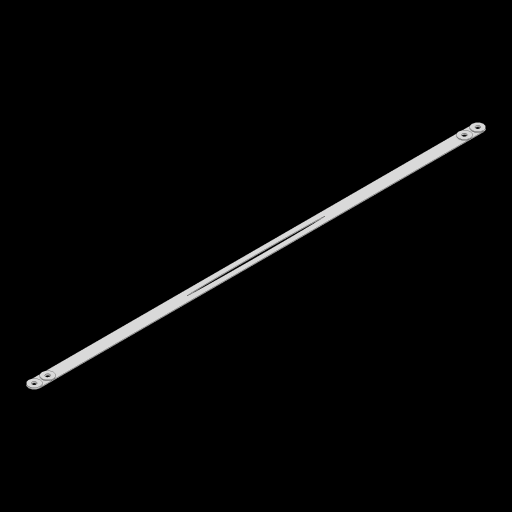
# Autodesk Inventor part: szalag4
Saved by Autodesk Inventor 2023 (Build 270158000, 158)
## iProperties
Created: 2022-11-17
Part Number: szalag4
Material: Generic
Document SubType Name: Modeling
Designer: gd1
Density: 1 g/cm^3
Appearance: Default
Author: gd1
Autodesk Inventor part; units mm, degrees
ref_plane "YZ Plane" through (0, 0, 0) normal (1, 0, 0) x (0, 1, 0)
ref_plane "XZ Plane" through (0, 0, 0) normal (0, 1, 0) x (-1, 0, 0)
ref_plane "XY Plane" through (0, 0, 0) normal (0, 0, 1) x (1, 0, 0)
sketch "Sketch1" plane through (0, 0, 0) normal (0, 1, 0) x (-1, 0, 0)
  line L0 (0, 0) -> (0, -273.901)
  line L1 (0, 0) -> (273.901, 0) construction
  line L2 (0, -273.901) -> (0, -319.801)
  line L3 (0, -319.801) -> (0, -593.702)
  line L4 (0, -319.801) -> (273.901, -319.801) construction
  line L5 (0, 0) -> (0, -15)
  line L6 (0, -593.702) -> (0, -578.702)
  circle A0 centre (0, -7.5) radius 7.5
  circle A1 centre (0, -586.202) radius 7.5
  line L7 (7.5, -7.5) -> (7.5, -586.202)
  line L8 (-7.5, -586.202) -> (-7.5, -7.5)
  line L9 (0, -15) -> (0, -17.5)
  line L10 (0, -17.5) -> (0, -32.5)
  circle A2 centre (0, -25) radius 7.5
  line L11 (-7.5, -296.851) -> (7.5, -296.851)
  circle A3 centre (0, -568.702) radius 7.5
  circle A4 centre (0, -7.5) radius 2.75
  circle A5 centre (0, -25) radius 2.75
  circle A6 centre (0, -586.202) radius 2.75
  circle A7 centre (0, -568.702) radius 2.75
  ellipse E0 centre (0, -296.851) end of major axis (0, -206.9528) minor radius 1.5
  line L12 (1.5, -296.851) -> (-1.5, -296.851)
  point P0 (-7.5, -568.702)
  point P1 (7.5, -568.702)
  point P2 (-7.5, -25)
  point P3 (7.5, -25)
  dimension "d0" = 273.901
  dimension "d1" = 90
  dimension "d2" = 45.9
  dimension "d3" = 273.901
  dimension "d4" = 90
  dimension "d5" = 15
  dimension "d6" = 15
  dimension "d7" = 2.5
  dimension "d8" = 15
  dimension "d9" = 5.5
  dimension "d10" = 5.5
  dimension "d15" = 3
  constraints: 26 end point, 8 centre point, 6 midpoint, 6 point on circle, 6 point on line, 3 symmetric about line, 3 tangent, 3 vertical, 2 coincident, 2 horizontal, 2 perpendicular, 7 other
  measures "d0" distance of L0.start L0.end
  measures "d1" angle of L0 L1
  measures "d2" distance of L0.end L2.end
  measures "d3" distance of L2.end L3.end
  measures "d4" angle of L3 L4
  measures "d5" distance of L0.start L5.end
  measures "d6" distance of L3.end L6.end
  measures "d7" distance of L5.end L9.end
  measures "d8" distance of L9.end L10.end
  measures "d9" diameter of A4
  measures "d10" diameter of A5
  measures "d15" distance of L12.start L12.end
extrude "Extrusion1" add sketch "Sketch1" along normal blind 1 contours A0 L7 A2 L0 | L0 A2 L8 A0 | L7 L11 E0 L0 A2 | A2 L0 E0 L11 L8 | L7 A3 L3 E0 L11 | L11 E0 L3 A3 L8 | L7 A1 L3 A3 | A3 L3 A1 L8
extrude "Extrusion2" add sketch "Sketch1" along normal blind 2 contours A0 L0 A4 | L0 A4 A0 | A2 L0 A5 | L0 A5 A2 | A3 L3 A7 | A3 L3 A7 | A1 L3 A6 | A1 L3 A6
body "Solid1"
